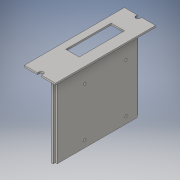
# Autodesk Inventor part: Slot
Saved by Autodesk Inventor 2016 (Build 200138000, 138)
## iProperties
Created: 2018-07-17
Part Number: Slot
Material: Generic
Document SubType Name: Modeling
Designer: Jorian Bruslind
Density: 1 g/cm^3
Appearance: Default
Author: Jorian Bruslind
Autodesk Inventor part; units mm, degrees
ref_plane "YZ Plane" through (0, 0, 0) normal (1, 0, 0) x (0, 1, 0)
ref_plane "XZ Plane" through (0, 0, 0) normal (0, 1, 0) x (-1, 0, 0)
ref_plane "XY Plane" through (0, 0, 0) normal (0, 0, 1) x (1, 0, 0)
sketch "Sketch1" plane through (0, 0, 0) normal (0, 1, 0) x (-1, 0, 0)
  line L0 (0, 0) -> (37, 0)
  line L1 (37, 0) -> (37, -119)
  line L2 (37, -119) -> (0, -119)
  line L3 (0, -119) -> (0, 0)
  dimension "d0" = 37
  dimension "d1" = 119
  constraints: 8 end point, 2 parallel, 1 horizontal, 1 perpendicular
  measures "d0" distance of L1.end L2.end
  measures "d1" distance of L0.end L1.end
extrude "Extrusion1" add sketch "Sketch1" along normal blind 2
sketch "Sketch3" plane through (0, 0, 0) normal (0, -1, 0) x (1, 0, 0)
  line L0 (0, 0) -> (-16.5, 0)
  line L1 (-37, 0) -> (0, 0) projected
  line L2 (-19, 0) -> (-19, -2)
  arc A0 (-21.5, -2) -> (-16.5, -2) centre (-19, -2) ccw
  line L3 (0, 0) -> (0, -119) projected
  line L4 (0, -119) -> (-19, -119)
  line L5 (0, -119) -> (-37, -119) projected
  line L6 (-19, -119) -> (-19, -117)
  arc A1 (-16.5, -117) -> (-21.5, -117) centre (-19, -117) ccw
  line L7 (-16.5, -117) -> (-16.5, -119)
  line L8 (-21.5, -117) -> (-21.5, -119)
  line L9 (-21.5, -119) -> (-16.5, -119)
  line L10 (-21.5, -2) -> (-21.5, 0)
  line L11 (-16.5, -2) -> (-16.5, 0)
  line L12 (-21.5, 0) -> (-16.5, 0)
  dimension "d14" = 19
  dimension "d15" = 2
  dimension "d16" = 5
  dimension "d17" = 19
  dimension "d18" = 2
  dimension "d19" = 5
  constraints: 20 end point, 6 point on line, 5 perpendicular, 4 point on circle, 2 centre point, 2 coincident, 2 horizontal, 1 parallel, 1 tangent
  measures "d14" distance of L0.start L2.start
  measures "d15" distance of L2.start L2.end
  measures "d16" diameter of A0
  measures "d17" distance of L3.end L4.end
  measures "d18" distance of L4.end L6.end
  measures "d19" diameter of A1
extrude "Extrusion3" cut sketch "Sketch3" against normal blind 2
sketch "Sketch4" plane through (0, 2, 0) normal (0, 1, 0) x (1, 0, 0)
  line L0 (0, 119) -> (0, 0) projected
  line L1 (0, 0) -> (0, 10)
  line L2 (0, 10) -> (-6, 10)
  line L3 (-32, 10) -> (-32, 105)
  line L4 (-6, 105) -> (-6, 10)
  line L5 (-6, 10) -> (-12.1, 10)
  line L6 (-6, 105) -> (-10.2, 105)
  line L7 (-10.2, 105) -> (-12.1, 105)
  line L8 (-12.5, 105) -> (-12.5, 107.7)
  line L9 (-12.5, 107.7) -> (-10.2, 107.7)
  line L10 (-10.2, 107.7) -> (-10.2, 105)
  line L11 (-6, 10) -> (-8, 10)
  line L12 (-8, 10) -> (-8, 105)
  line L13 (-12.5, 105) -> (-12.5, 103)
  line L14 (-12.5, 103) -> (-10, 103)
  line L15 (-10, 103) -> (-10, 12)
  line L16 (-6, 10) -> (-12.1, 10)
  line L17 (-15.4, 10) -> (-32, 10)
  line L18 (-32, 105) -> (-12.5, 105)
  line L19 (-10.2, 105) -> (-6, 105)
  line L20 (-10, 12) -> (-12.5, 12)
  line L21 (-12.5, 12) -> (-12.5, 10)
  line L22 (-12.5, 10) -> (-12.5, 7.3)
  line L23 (-12.5, 7.3) -> (-10.2, 7.3)
  line L24 (-10.2, 7.3) -> (-10.2, 10)
  line L25 (-15.4, 10) -> (-12.5, 10)
  point P0 (-19, 2)
  dimension "d59" = 10
  dimension "d60" = 6
  dimension "d61" = 26
  dimension "d62" = 95
  dimension "d66" = 4.2
  dimension "d67" = 2.3
  dimension "d73" = 2
  dimension "d76" = 2.5
  dimension "d101" = 2.5
  dimension "d102" = 2.7
  dimension "d103" = 4.5
  dimension "d106" = 2
  dimension "d107" = 2.7
  dimension "d108" = 2
  dimension "d109" = 2
  dimension "d110" = 2
  constraints: 50 end point, 8 perpendicular, 7 horizontal, 7 parallel, 5 point on line, 1 vertical
  measures "d59" distance of L0.end L1.end
  measures "d60" distance of L1.end L2.end
  measures "d61" distance of L3.end L4.start
  measures "d62" distance of L3.start L3.end
  measures "d66" distance of L4.start L6.end
  measures "d67" distance of L8.end L9.end
  measures "d73" distance of L2.end L11.end
  measures "d76" distance of L13.end L14.end
  measures "d101" distance of L15.end L20.end
  measures "d102" distance of L21.end L22.end
  measures "d103" distance between parallel lines of L12 L22
  measures "d106" distance between parallel lines of L18 L14
  measures "d107" distance of L8.start L8.end
  measures "d108" distance between parallel lines of L6 L14
  measures "d109" distance between parallel lines of L20 L16
  measures "d110" distance between parallel lines of L25 L20
extrude "Extrusion7" add sketch "Sketch4" against normal blind 92 contours L8 L9 L10 L6 L12 L5 L24 L23 L22 L21 L20 L15 L14 L13 | L6 L4 L5 L12
sketch "Sketch6" plane through (-10, -90, -103) normal (-1, 0, 0) x (0, 0, 1)
  line L0 (103, 92) -> (-16, 92) projected
  line L1 (-4.7, 92) -> (60.3, 92)
  line L2 (60.3, 92) -> (60.3, 66.128)
  circle A0 centre (60.3, 66.128) radius 1.375
  line L3 (-4.7, 90) -> (-4.7, 0) projected
  line L4 (60.3, 66.128) -> (60.3, 8.128)
  circle A1 centre (60.3, 8.128) radius 1.375
  line L5 (60.3, 8.128) -> (11.3, 8.128)
  circle A2 centre (11.3, 8.128) radius 1.375
  line L6 (11.3, 8.128) -> (11.3, 66.128)
  circle A3 centre (11.3, 66.128) radius 1.375
  point P0 (103, 90)
  dimension "d16" = 5
  dimension "d80" = 65
  dimension "d81" = 25.872
  dimension "d82" = 2.75
  dimension "d83" = 65
  dimension "d87" = 58
  dimension "d88" = 2.75
  dimension "d89" = 49
  dimension "d90" = 2.75
  dimension "d91" = 2.75
  constraints: 10 end point, 4 centre point, 4 coincident, 2 point on line, 2 vertical, 1 horizontal, 1 perpendicular
  measures "d80" distance of L1.start L1.end
  measures "d81" distance of L1.end L2.end
  measures "d82" diameter of A0
  measures "d83" distance between parallel lines of L3 L2
  measures "d87" distance of L4.start L4.end
  measures "d88" diameter of A1
  measures "d89" distance of L5.start L5.end
  measures "d90" diameter of A2
  measures "d91" diameter of A3
extrude "Extrusion8" cut sketch "Sketch6" against normal blind 2
sketch "Sketch7" plane through (0, 0, 0) normal (0, -1, 0) x (1, 0, 0)
  line L0 (-10, -103) -> (-10, -12) projected
  line L1 (-10, -103) -> (-10, -41)
  line L2 (-10, -41) -> (-12.9, -41)
  line L3 (-12.9, -41) -> (-28.9, -41)
  line L4 (-28.9, -41) -> (-28.9, -95)
  line L5 (-28.9, -95) -> (-12.9, -95)
  line L6 (-12.9, -95) -> (-12.9, -41)
  point P0 (0, 0)
  dimension "d94" = 62
  dimension "d95" = 2.9
  dimension "d96" = 16
  dimension "d97" = 54
  constraints: 12 end point, 2 horizontal, 2 parallel, 1 perpendicular, 1 point on line
  measures "d94" distance of L0.start L1.end
  measures "d95" distance of L1.end L2.end
  measures "d96" distance of L5.end L4.end
  measures "d97" distance of L4.end L3.end
extrude "Extrusion9" cut sketch "Sketch7" against normal blind 2
sketch "Sketch8" plane through (-6, -90, -10) normal (1, 0, 0) x (0, 0, -1)
  line L0 (0, 90) -> (0, 0) projected
  line L1 (95, 90) -> (95, 0) projected
  line L2 (0, 0) -> (95, 0)
  line L3 (95, 0) -> (95, 90)
  line L4 (95, 90) -> (0, 90)
  line L5 (0, 90) -> (0, 0)
  point P0 (-10, 90)
  constraints: 8 end point, 2 parallel, 1 horizontal, 1 perpendicular
extrude "Extrusion10" cut sketch "Sketch8" against normal blind 2
body "Solid1"
